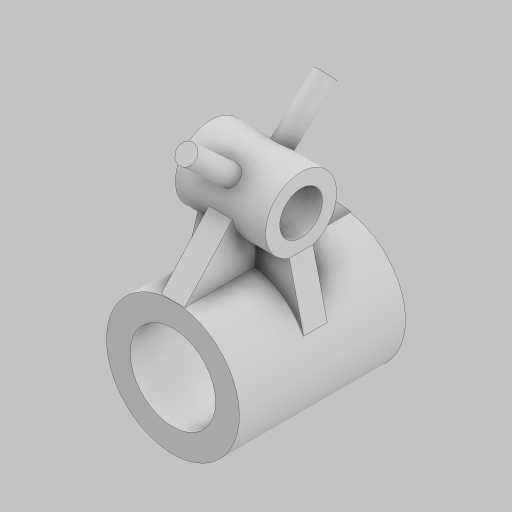
# Autodesk Inventor part: parte_1
Saved by Autodesk Inventor 2023 (Build 270158000, 158)
## iProperties
Created: 2022-08-24
Part Number: parte_1
Material: Generic
Document SubType Name: Modeling
Designer: river
Density: 1 g/cm^3
Appearance: Default
Author: river
Autodesk Inventor part; units mm, degrees
ref_plane "YZ Plane" through (0, 0, 0) normal (1, 0, 0) x (0, 1, 0)
ref_plane "XZ Plane" through (0, 0, 0) normal (0, 1, 0) x (-1, 0, 0)
ref_plane "XY Plane" through (0, 0, 0) normal (0, 0, 1) x (1, 0, 0)
sketch "Sketch6" plane through (0, 0, 0) normal (0, 0, 1) x (1, 0, 0)
  circle A0 centre (0, 0) radius 9
  circle A1 centre (0, 0) radius 14
  dimension "d20" = 18
  dimension "d21" = 28
  constraints: 2 centre point, 2 coincident
  measures "d20" diameter of A0
  measures "d21" diameter of A1
extrude "Extrusion4" add sketch "Sketch6" along normal blind 35
ref_plane "Work Plane2" through (0, 0, 17.5) normal (0, 0, 1) x (1, 0, 0)
sketch "Sketch8" plane through (0, 0, 17.5) normal (0, 0, 1) x (1, 0, 0)
  line L0 (0, 0) -> (0, 26)
  line L1 (0, 26) -> (-9.5, 26)
  line L2 (-9.5, 26) -> (-9.5, 21.5)
  line L3 (-9.5, 21.5) -> (0, 21.5)
  line L4 (0, 21.5) -> (0, 26)
  line L5 (0, 21.5) -> (-9.5, 21.5)
  line L6 (-9.5, 21.5) -> (-9.5, 18.5)
  line L7 (-9.5, 18.5) -> (0, 18.5)
  line L8 (0, 18.5) -> (0, 21.5)
  line L9 (9.5, 21.5) -> (0, 21.5)
  line L10 (9.5, 21.5) -> (9.5, 18.5)
  line L11 (9.5, 18.5) -> (0, 18.5)
  dimension "d28" = 26
  dimension "d29" = 9.5
  dimension "d30" = 4.5
  dimension "d32" = 3
  constraints: 24 end point, 4 parallel, 3 symmetric about line, 2 horizontal, 2 perpendicular, 1 vertical
  measures "d28" distance of L0.start L0.end
  measures "d29" distance of L3.end L2.end
  measures "d30" distance of L2.end L1.end
  measures "d32" distance of L5.end L6.end
revolve "Revolution1" add sketch "Sketch8" angle 360 about axis through (0, 26, 17.5) along (-1, 0, 0) contours L7 L6 L3 L0 | L0 L9 L10 L11
sketch "Sketch10" plane through (0, 0, 17.5) normal (0, 0, 1) x (1, 0, 0)
  circle A0 centre (0, 0) radius 14 projected
  line L0 (-14, 0) -> (-9.5, 19)
  line L1 (-9.5, 19) -> (0, 19)
  line L2 (-9.5, 33.5) -> (-9.5, 18.5) projected
  line L3 (0, 19) -> (0, 0)
  line L4 (14, 0) -> (9.5, 19)
  line L5 (9.5, 19) -> (0, 19)
  point P0 (-12.5128, 6.2793)
  point P1 (12.5128, 6.2793)
  dimension "d35" = 19
  dimension "d36" = 9.5
  constraints: 10 end point, 2 perpendicular, 2 symmetric about line, 2 other
  measures "d35" distance of L1.end L3.end
  measures "d36" distance of L4.end L1.end
extrude "Extrusion6" add sketch "Sketch10" along normal blind 2.5 contours L0 L1 L3 A0 | A0 L3 L5 L4
mirror "Mirror2" about plane through (0, 0, 17.5) normal (0, 0, 1) of "Extrusion6"
ref_plane "Work Plane3" through (0, 59.1111, 15) normal (-1, 0, 0) x (0, 0, 1)
sketch "Sketch11" plane through (0, 59.1111, 15) normal (-1, 0, 0) x (0, 0, 1)
  arc A0 (5, -40.1822) -> (0, -40.1822) centre (2.5, -33.1111) ccw projected
  line L0 (-4.9336, -34.1072) -> (-15, -45.1111)
  line L1 (-15, -45.1111) -> (20, -45.1111) projected
  circle A1 centre (2.5, -33.1111) radius 7.5
  line L2 (2.5, -33.1111) -> (2.5, -59.6944)
  line L3 (10, -34.1161) -> (20, -45.1111)
  point P0 (-15, -59.1111)
  point P1 (10, -33.1111)
  point P2 (2.5, -45.1111)
  point P3 (2.5, -40.6111)
  constraints: 6 end point, 1 centre point, 1 coincident, 1 concentric, 1 point on circle, 1 point on line, 1 symmetric about line, 1 vertical
extrude "Extrusion9" add sketch "Sketch11" along normal blind 2.5 contours L2 L1 L0 A0 A1
mirror "Mirror5" about plane through (0, 59.1111, 15) normal (-1, 0, 0) of "Extrusion9"
mirror "Mirror6" about plane through (0, 0, 17.5) normal (0, 0, 1) of "Extrusion9", "Mirror5"
sketch "Sketch13" plane through (2.5, 25.0039, 10.0664) normal (0, 0.675, -0.7378) x (-1, 0, 0)
  line L0 (0, 0) -> (5, 0) projected
  line L1 (0, 0) -> (5, 0)
  line L2 (5, 0) -> (5, 11.3934)
  line L3 (5, 11.3934) -> (0, 11.3934)
  line L4 (0, 11.3934) -> (0, 0)
  line L5 (0, 11.3934) -> (5, 0)
  line L6 (0, 0) -> (5, 11.3934)
  line L7 (2.5, -1.4142) -> (2.5, 8.7105) projected
  circle A0 centre (2.5, 5.6967) radius 2.0284
  point P0 (2.5, -25.2434)
  constraints: 12 end point, 2 parallel, 1 centre point, 1 horizontal, 1 midpoint, 1 perpendicular, 1 point on line
extrude "Extrusion10" add sketch "Sketch13" along normal blind 15 contours A0 L5 L6 | L6 L7 A0 | L7 L5 A0 | A0 L7 L5 | L6 A0 L5 | L7 A0 L6
mirror "Mirror7" about plane through (0, 0, 17.5) normal (0, 0, 1) of "Extrusion10"
body "Solid2"
